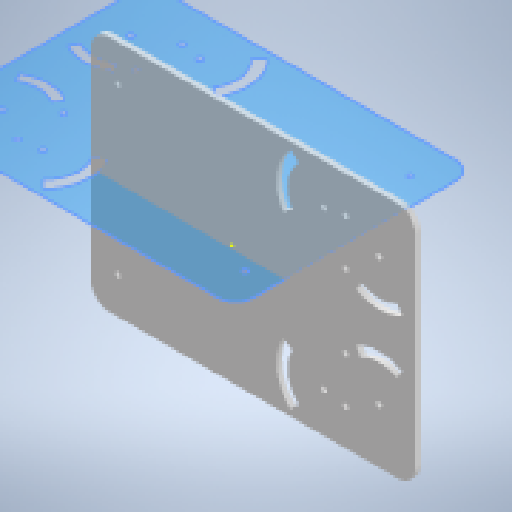
# Autodesk Inventor part: Middle layer
Saved by Autodesk Inventor 2023 (Build 270158000, 158)
## iProperties
Created: 2024-10-04
Part Number: Middle layer
Material: Generic
Document SubType Name: Modeling
Designer: bw1293
Density: 1 g/cm^3
Appearance: Default
Author: bw1293
Autodesk Inventor part; units mm, degrees
ref_plane "YZ Plane" through (0, 0, 0) normal (1, 0, 0) x (0, 1, 0)
ref_plane "XZ Plane" through (0, 0, 0) normal (0, 1, 0) x (-1, 0, 0)
ref_plane "XY Plane" through (0, 0, 0) normal (0, 0, 1) x (1, 0, 0)
sketch "Sketch1" plane through (0, 0, 0) normal (0, 0, 1) x (1, 0, 0)
  line L0 (100, 55) -> (100, -55)
  line L1 (-100, 65) -> (100, -65) construction
  line L2 (100, 65) -> (-100, -65) construction
  circle A0 centre (61.75, -20) radius 1.5
  circle A1 centre (61.75, 20) radius 1.5
  circle A2 centre (-62.75, -45) radius 1.5
  circle A3 centre (-62.75, 45) radius 1.5
  arc A4 (100, 55) -> (90, 65) centre (90, 55) ccw
  arc A5 (90, -65) -> (100, -55) centre (90, -55) ccw
  circle A6 centre (61.75, 45) radius 1.5
  circle A7 centre (61.75, -45) radius 1.5
  line L3 (-77.5, 55) -> (-77.5, -55)
  arc A8 (-67.5, 65) -> (-77.5, 55) centre (-67.5, 55) ccw
  arc A9 (-77.5, -55) -> (-67.5, -65) centre (-67.5, -55) ccw
  line L4 (-67.5, 65) -> (90, 65)
  line L5 (90, -65) -> (-67.5, -65)
  point P0 (0, 0)
extrude "Extrusion1" add sketch "Sketch1" along normal blind 3
sketch "Sketch2" plane through (0, 0, 3) normal (0, 0, 1) x (1, 0, 0)
  line L0 (100, -55) -> (100, 55) projected
  line L1 (90, 65) -> (-90, 65) projected
  arc A0 (100, 55) -> (90, 65) centre (90, 55) ccw projected
  arc A1 (90, -65) -> (100, -55) centre (90, -55) ccw projected
  line L2 (-90, -65) -> (90, -65) projected
  arc A2 (-100, -55) -> (-90, -65) centre (-90, -55) ccw projected
  line L3 (-100, 55) -> (-100, -55) projected
  arc A3 (-90, 65) -> (-100, 55) centre (-90, 55) ccw projected
  line L4 (100, 0) -> (-100, 0)
  line L5 (0, -65) -> (0, 65)
  line L6 (100, 0) -> (80, 0)
  line L7 (80, 0) -> (80, -35)
  circle A4 centre (80, -35) radius 1.5
  line L8 (80, -35) -> (80, -12.5)
  line L9 (82.6, -15.1) -> (77.4, -15.1)
  line L10 (77.4, -15.1) -> (77.4, -9.9)
  line L11 (77.4, -9.9) -> (82.6, -9.9)
  line L12 (82.6, -9.9) -> (82.6, -15.1)
  line L13 (82.6, -15.1) -> (77.4, -9.9) construction
  line L14 (77.4, -15.1) -> (82.6, -9.9) construction
  arc A5 (80, -12.5) -> (68.75, -15.5144) centre (80, -35) ccw construction
  arc A6 (80, -9.9) -> (67.45, -13.2628) centre (80, -35) ccw
  arc A7 (80, -15.1) -> (70.05, -17.7661) centre (80, -35) ccw
  line L15 (80, -35) -> (68.75, -15.5144) construction
  line L16 (80, -35) -> (80, -12.5) construction
  arc A8 (91.25, -15.5144) -> (80, -12.5) centre (80, -35) ccw construction
  arc A9 (92.55, -13.2628) -> (80, -9.9) centre (80, -35) ccw
  arc A10 (89.95, -17.7661) -> (80, -15.1) centre (80, -35) ccw
  line L17 (80, -35) -> (91.25, -15.5144) construction
  line L18 (80, -35) -> (80, -12.5) construction
  line L19 (70.05, -17.7661) -> (67.45, -13.2628)
  line L20 (89.95, -17.7661) -> (92.55, -13.2628)
  circle A11 centre (80, 35) radius 1.5
  arc A12 (67.45, 13.2628) -> (80, 9.9) centre (80, 35) ccw
  arc A13 (70.05, 17.7661) -> (80, 15.1) centre (80, 35) ccw
  arc A14 (80, 9.9) -> (92.55, 13.2628) centre (80, 35) ccw
  arc A15 (80, 15.1) -> (89.95, 17.7661) centre (80, 35) ccw
  line L21 (70.05, 17.7661) -> (67.45, 13.2628)
  line L22 (89.95, 17.7661) -> (92.55, 13.2628)
  line L23 (100, 55) -> (50, 55)
  line L24 (50, 55) -> (50, 65)
  line L25 (50, 55) -> (50, 43)
  circle A16 centre (50, 43) radius 1.5
  line L26 (50, 43) -> (30.075, 43)
  line L27 (23.875, 39.85) -> (30.075, 39.85)
  line L28 (30.075, 39.85) -> (30.075, 43)
  line L29 (23.875, 46.15) -> (30.075, 46.15)
  line L30 (30.075, 46.15) -> (30.075, 43)
  line L31 (23.875, 46.15) -> (23.875, 39.85)
  arc A17 (33.7189, 59.2811) -> (26.975, 43) centre (50, 43) ccw construction
  arc A18 (31.5268, 61.4732) -> (23.875, 43) centre (50, 43) ccw
  arc A19 (35.9109, 57.0891) -> (30.075, 43) centre (50, 43) ccw
  line L32 (50, 43) -> (33.7189, 59.2811) construction
  line L33 (50, 43) -> (26.975, 43) construction
  arc A20 (26.975, 43) -> (30.0598, 31.4875) centre (50, 43) ccw construction
  arc A21 (23.875, 43) -> (27.3751, 29.9375) centre (50, 43) ccw
  arc A22 (30.075, 43) -> (32.7444, 33.0375) centre (50, 43) ccw
  line L34 (50, 43) -> (30.0598, 31.4875) construction
  line L35 (50, 43) -> (26.975, 43) construction
  line L36 (35.9109, 57.0891) -> (31.5268, 61.4732)
  line L37 (32.7444, 33.0375) -> (27.3751, 29.9375)
  circle A23 centre (27.108, 7.5) radius 1.5 projected
  circle A24 centre (-20.392, 55) radius 1.5 projected
  circle A25 centre (-67.892, 7.5) radius 1.5 projected
  circle A26 centre (27.108, 7.5) radius 1.5
  circle A27 centre (-20.392, 55) radius 1.5
  circle A28 centre (-67.892, 7.5) radius 1.5
  circle A29 centre (50, -43) radius 1.5
  arc A30 (23.875, -43) -> (31.5268, -61.4732) centre (50, -43) ccw
  arc A31 (30.075, -43) -> (35.9109, -57.0891) centre (50, -43) ccw
  arc A32 (27.3751, -29.9375) -> (23.875, -43) centre (50, -43) ccw
  arc A33 (32.7444, -33.0375) -> (30.075, -43) centre (50, -43) ccw
  line L38 (35.9109, -57.0891) -> (31.5268, -61.4732)
  line L39 (32.7444, -33.0375) -> (27.3751, -29.9375)
  point P0 (0, 0)
  point P1 (80, -15.1)
  point P2 (80, -9.9)
  point P3 (23.875, 43)
  point P4 (23.875, -43)
  dimension "d7" = 20
  dimension "d8" = 35
  dimension "d9" = 3
  dimension "d10" = 22.5
  dimension "d11" = 5.2
  dimension "d12" = 5.2
  dimension "d13" = 30
  dimension "d15" = 30
  dimension "d17" = 50
  dimension "d18" = 12
  dimension "d19" = 3
  dimension "d20" = 19.925
  dimension "d21" = 6.2
  dimension "d23" = 6.2
  dimension "d25" = 6.3
  dimension "d26" = 45
  dimension "d28" = 30
  dimension "d32" = 3
  dimension "d33" = 3
  dimension "d34" = 3
  constraints: 72 end point, 44 point on circle, 27 centre point, 24 symmetric about line, 13 coincident, 6 midpoint, 5 point on line, 3 horizontal, 2 collinear, 2 concentric, 2 parallel, 2 perpendicular, 2 vertical, 10 other
  measures "d7" distance of L4.start L6.end
  measures "d8" distance of L6.end L7.end
  measures "d9" diameter of A4
  measures "d10" distance of L8.start L8.end
  measures "d11" distance of L10.end L11.end
  measures "d12" distance of L9.end L10.end
  measures "d13" angle of L16 L15
  measures "d15" angle of L17 L18
  measures "d17" distance of L0.end L23.end
  measures "d18" distance of L23.end L25.end
  measures "d19" diameter of A16
  measures "d20" distance of L26.start L26.end
  measures "d21" distance of L27.end L27.start
  measures "d23" distance of L29.start L29.end
  measures "d25" distance of L29.start L27.start
  measures "d26" angle of L32 L33
  measures "d28" angle of L35 L34
  measures "d32" diameter of A26
  measures "d33" diameter of A27
  measures "d34" diameter of A28
sketch "Sketch4" plane through (0, 0, 3) normal (0, 0, 1) x (1, 0, 0)
  point P0 (0, 0)
extrude "Extrusion7" cut sketch "Sketch2" against normal blind 10 contours A9 L12 L9 L7 | L7 L9 L10 A6 | L10 L9 A7 L19 A6 | A9 L20 A10 L9 L12 | A4 | A11 | L21 A13 A15 L22 A14 A12 | A16 L26 L25 | L25 L26 A16 | A21 A18 L29 L30 L28 L27 | L27 L28 A22 L37 A21 | A18 L36 A19 L30 L29 | A29 | A32 L39 A33 A31 L38 A30
body "Solid1"
